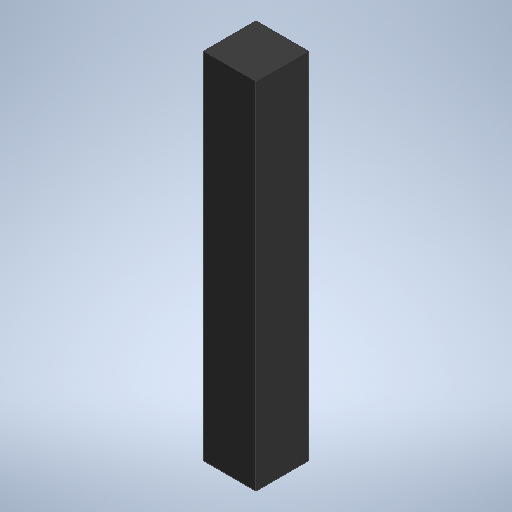
# Autodesk Inventor part: CableFemale
Saved by Autodesk Inventor 2025.1 (Build 291241020, 241B)
## iProperties
Created: 2024-09-01
Part Number: CableFemale
Material: Generic
Document SubType Name: Modeling
Designer: andre
Density: 1 g/cm^3
Appearance: Default
Author: andre
Autodesk Inventor part; units mm, degrees
ref_plane "YZ Plane" through (0, 0, 0) normal (1, 0, 0) x (0, 1, 0)
ref_plane "XZ Plane" through (0, 0, 0) normal (0, 1, 0) x (-1, 0, 0)
ref_plane "XY Plane" through (0, 0, 0) normal (0, 0, 1) x (1, 0, 0)
sketch "Sketch1" plane through (0, 0, 0) normal (0, 1, 0) x (-1, 0, 0)
  line L0 (0, 0) -> (2.8, 0)
  line L1 (2.8, 0) -> (2.8, -2.8)
  line L2 (2.8, -2.8) -> (0, -2.8)
  line L3 (0, -2.8) -> (0, 0)
  line L4 (1.8, -1.8) -> (1, -1.8)
  line L5 (1, -1.8) -> (1, -1)
  line L6 (1, -1) -> (1.8, -1)
  line L7 (1.8, -1) -> (1.8, -1.8)
  point P0 (1.4, -1)
  point P1 (1.4, 0)
  point P2 (1.8, -1.4)
  point P3 (2.8, -1.4)
  dimension "d0" = 2.8
  dimension "d1" = 2.8
  dimension "d2" = 0.8
  dimension "d3" = 0.8
  constraints: 16 end point, 4 midpoint, 4 parallel, 2 horizontal, 2 perpendicular, 1 horizontal alignment, 1 vertical alignment
  measures "d0" distance of L1.end L2.end
  measures "d1" distance of L0.end L1.end
  measures "d2" distance of L5.end L6.end
  measures "d3" distance of L4.end L5.end
extrude "Extrusion1" add sketch "Sketch1" along normal blind 19
sketch "Sketch2" plane through (0, 19, 0) normal (0, 1, 0) x (1, 0, 0)
  line L0 (-1.8, 1) -> (-1.8, 1.8) projected
  line L1 (0, 2.8) -> (-2.8, 2.8) projected
  line L2 (-2.8, 2.8) -> (-2.8, 0) projected
  line L3 (-2.8, 0) -> (0, 0) projected
  line L4 (0, 0) -> (0, 2.8) projected
  line L5 (-1.8, 1.8) -> (-1, 1.8) projected
  line L6 (-1, 1.8) -> (-1, 1) projected
  line L7 (-1, 1) -> (-1.8, 1) projected
  line L8 (-1.8, 1) -> (-1.8, 1.8) projected
extrude "Extrusion2" add sketch "Sketch2" against normal blind 2 contours L0 L5 L6 L7
body "Solid1"
